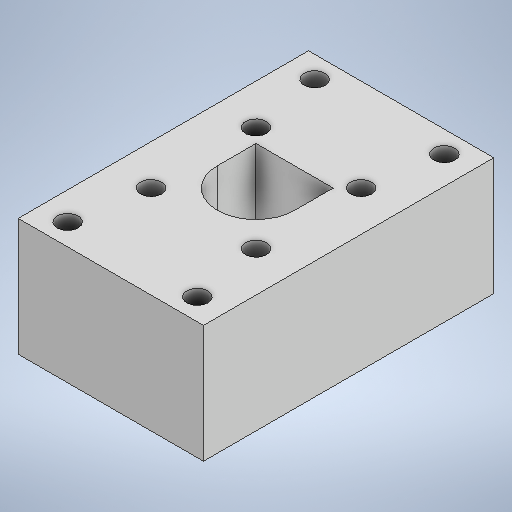
# Autodesk Inventor part: HopefullyHelpsMount
Saved by Autodesk Inventor 2027 (Build 310192060, 192F)
## iProperties
Created: 2026-07-07
Part Number: HopefullyHelpsMount
Material: Generic
Document SubType Name: Modeling
Designer: 13129
Density: 1 g/cm^3
Appearance: Default
Author: 13129
Autodesk Inventor part; units mm, degrees
ref_plane "YZ Plane" through (0, 0, 0) normal (1, 0, 0) x (0, 1, 0)
ref_plane "XZ Plane" through (0, 0, 0) normal (0, 1, 0) x (-1, 0, 0)
ref_plane "XY Plane" through (0, 0, 0) normal (0, 0, 1) x (1, 0, 0)
sketch "Sketch1" plane through (0, 0, 0) normal (0, 1, 0) x (-1, 0, 0)
  line L0 (0, 0) -> (0, 47)
  line L1 (0, 47) -> (30, 47)
  line L2 (30, 47) -> (30, 0)
  line L3 (30, 0) -> (0, 0)
  dimension "d0" = 47
  dimension "d1" = 30
  constraints: 8 end point, 3 perpendicular, 1 vertical
  measures "d0" distance of L0.start L0.end
  measures "d1" distance of L0.end L1.end
extrude "Extrusion1" add sketch "Sketch1" along normal blind 19.05
sketch "Sketch2" plane through (0, 19.05, 0) normal (0, 1, 0) x (1, 0, 0)
  line L0 (-30, 0) -> (-30, -47) construction
  line L1 (0, 0) -> (-30, 0) construction
  circle A0 centre (-25.5, -43.5) radius 1.7
  circle A1 centre (-4.5, -43.5) radius 1.7
  circle A2 centre (-23.5, -32) radius 1.7
  circle A3 centre (-6.5, -32) radius 1.7
  circle A4 centre (-23.5, -15) radius 1.7
  circle A5 centre (-25.5, -3.5) radius 1.7
  circle A6 centre (-4.5, -3.5) radius 1.7
  circle A7 centre (-6.5, -15) radius 1.7
  line L2 (-23.5, -32) -> (-23.5, -15)
  line L3 (-23.5, -15) -> (-6.5, -15)
  line L4 (-25.5, -43.5) -> (-25.5, -3.5)
  line L5 (-25.5, -3.5) -> (-4.5, -3.5)
  circle A8 centre (-15, -23.5) radius 6.25
  line L6 (-21.25, -23.5) -> (-21.25, -17.25)
  line L7 (-21.25, -17.25) -> (-8.75, -17.25)
  line L8 (-8.75, -17.25) -> (-8.75, -23.5)
  point P0 (-25.5, -23.5)
  point P1 (-30, -23.5)
  point P2 (-23.5, -23.5)
  point P3 (-30, -23.5)
  point P4 (-15, -3.5)
  point P5 (-15, 0)
  point P6 (-15, -15)
  point P7 (-15, 0)
  point P8 (-15, 0)
  point P9 (-30, -23.5)
  point P10 (-15, -17.25)
  dimension "d4" = 3.4
  dimension "d5" = 17
  dimension "d6" = 17
  dimension "d7" = 40
  dimension "d8" = 21
  dimension "d9" = 12.5
  constraints: 14 end point, 10 midpoint, 9 centre point, 7 equal radius, 7 horizontal alignment, 7 vertical alignment, 4 perpendicular, 3 tangent, 3 vertical, 2 point on circle
  measures "d4" diameter of A2
  measures "d5" distance of L2.start L2.end
  measures "d6" distance of L2.end L3.end
  measures "d7" distance of L4.start L4.end
  measures "d8" distance of L4.end L5.end
  measures "d9" diameter of A8
extrude "Extrusion2" cut sketch "Sketch2" against normal through all
body "Solid1"
